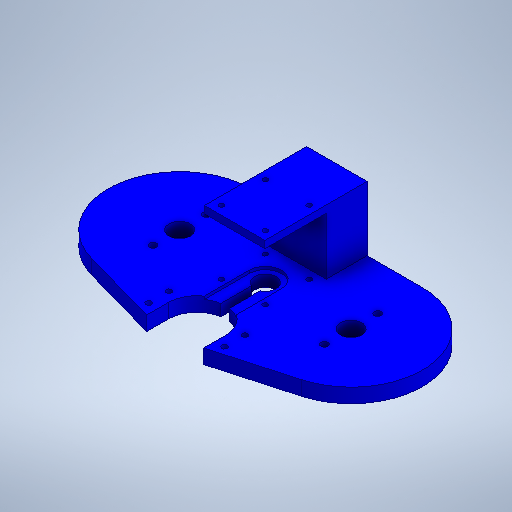
# Autodesk Inventor part: ExtruderFrame
Saved by Autodesk Inventor 2025.2 (Build 292293000, 293)
## iProperties
Created: 2025-05-30
Part Number: ExtruderFrame
Material: Generic
Document SubType Name: Modeling
Designer: Simon
Density: 1 g/cm^3
Appearance: Default(2)
Author: Simon
Autodesk Inventor part; units mm, degrees
ref_plane "YZ Plane" through (0, 0, 0) normal (1, 0, 0) x (0, 1, 0)
ref_plane "XZ Plane" through (0, 0, 0) normal (0, 1, 0) x (-1, 0, 0)
ref_plane "XY Plane" through (0, 0, 0) normal (0, 0, 1) x (1, 0, 0)
sketch "Sketch6" plane through (0, 0, 0) normal (0, 1, 0) x (-1, 0, 0)
  line L0 (60, 0) -> (-60, 0)
  circle A0 centre (0, 0) radius 30
  circle A1 centre (-60, 0) radius 50
  circle A2 centre (60, 0) radius 50
  circle A3 centre (60, 0) radius 7.5
  circle A4 centre (0, 0) radius 7.5
  circle A5 centre (-60, 0) radius 7.5
  line L1 (60, -50) -> (-60, -50)
  line L2 (-60, 18.65) -> (-60, -18.65)
  line L3 (60, 18.65) -> (60, -18.65)
  line L4 (0, -15.3795) -> (0, 15.3795)
  line L5 (15.3795, 15.3795) -> (-15.3795, 15.3795)
  line L6 (15.3795, -15.3795) -> (-15.3795, -15.3795)
  line L7 (21.15, 21.5) -> (-21.15, 21.5)
  line L8 (-21.15, 21.5) -> (-21.15, -21.5)
  line L9 (-21.15, -21.5) -> (21.15, -21.5)
  line L10 (21.15, -21.5) -> (21.15, 21.5)
  line L11 (21.15, 21.5) -> (-21.15, -21.5) construction
  line L12 (-21.15, 21.5) -> (21.15, -21.5) construction
  line L13 (21.15, -21.5) -> (-21.15, -21.5)
  line L14 (-21.15, -21.5) -> (-21.15, -50)
  line L15 (-21.15, -50) -> (21.15, -50)
  line L16 (21.15, -50) -> (21.15, -21.5)
  line L17 (7.5, 0) -> (-7.7, 0)
  line L18 (-7.7, 0) -> (-7.7, 50)
  line L19 (-7.7, 50) -> (7.5, 50)
  line L20 (7.5, 50) -> (7.5, 0)
  line L21 (3, -100) -> (-3, -100)
  line L22 (-3, -100) -> (-3, 100)
  line L23 (-3, 100) -> (3, 100)
  line L24 (3, 100) -> (3, -100)
  line L25 (3, -100) -> (-3, 100) construction
  line L26 (-3, -100) -> (3, 100) construction
  line L27 (11.25, 100) -> (-11.25, 100)
  line L28 (-11.25, 100) -> (-11.25, -100)
  line L29 (-11.25, -100) -> (11.25, -100)
  line L30 (11.25, -100) -> (11.25, 100)
  line L31 (11.25, 100) -> (-11.25, -100) construction
  line L32 (-11.25, 100) -> (11.25, -100) construction
  circle A6 centre (0, 0) radius 11.25
  line L33 (0, 0) -> (0, 48)
  circle A7 centre (0, 48) radius 20
  line L34 (73.5118, 48.1397) -> (5.4047, 67.2559)
  line L35 (-73.5118, 48.1397) -> (-5.4047, 67.2559)
  line L36 (-20, 48) -> (20, 48)
  line L37 (20, 48) -> (20, 63.1593)
  line L38 (-20, 48) -> (-20, 63.1593)
  circle A8 centre (0, 48) radius 27.5
  line L39 (0, 48) -> (-26.563, 40.8825)
  line L40 (0, 48) -> (27.5, 48) construction
  line L41 (0, 48) -> (-26.563, 55.1175)
  line L42 (0, 48) -> (26.563, 40.8825)
  line L43 (0, 48) -> (26.563, 55.1175)
  point P0 (16.6667, 24.9444)
  point P1 (-16.6667, 24.9444)
  point P2 (-7.5, 0)
  point P3 (-3, 0)
  point P4 (3, 0)
  point P5 (-21.15, -21.5)
  point P6 (21.15, -50)
  point P7 (11.25, 0)
  point P8 (3, 100)
  point P9 (-11.25, 0)
  point P10 (-11.25, 65.6152)
  point P11 (-7.7, 28.995)
  point P12 (-7.7, 29.5417)
  point P13 (-11.25, 64.5359)
  point P14 (11.25, 65.6152)
  point P15 (11.25, 64.5359)
  point P16 (7.5, 29.4595)
  point P17 (7.5, 29.0474)
  point P18 (-6.8464, 29.2083)
  point P19 (6.8464, 29.2083)
  dimension "d42" = 15
  dimension "d37" = 120
  dimension "d38" = 60
  dimension "d39" = 100
  dimension "d40" = 100
  dimension "d41" = 15
  dimension "d43" = 15
  dimension "d46" = 37.3
  dimension "d47" = 37.3
  dimension "d48" = 30.759
  dimension "d49" = 30.759
  dimension "d50" = 30.759
  dimension "d65" = 42.3
  dimension "d66" = 43
  dimension "d67" = 50
  dimension "d70" = 6
  dimension "d71" = 200
  dimension "d76" = 22.5
  dimension "d77" = 200
  dimension "d93" = 48
  dimension "d94" = 40
  dimension "d97" = 55
  dimension "d98" = 165
  constraints: 88 end point, 14 midpoint, 13 parallel, 11 point on circle, 8 centre point, 8 coincident, 7 perpendicular, 6 horizontal, 6 tangent, 5 point on line, 4 vertical, 1 equal length, 3 other
  measures "d37" distance of L0.start L0.end
  measures "d38" diameter of A0
  measures "d39" diameter of A1
  measures "d40" diameter of A2
  measures "d41" diameter of A3
  measures "d43" diameter of A5
  measures "d46" distance of L2.start L2.end
  measures "d47" distance of L3.start L3.end
  measures "d48" distance of L4.start L4.end
  measures "d49" distance of L5.start L5.end
  measures "d50" distance of L6.start L6.end
  measures "d65" distance of L9.end L8.end
  measures "d66" distance of L8.end L7.end
  measures "d67" distance of L17.end L18.end
  measures "d70" distance of L21.start L21.end
  measures "d71" distance of L21.end L22.end
  measures "d76" distance of L27.start L27.end
  measures "d77" distance of L28.end L27.end
  measures "d93" distance of L33.start L33.end
  measures "d94" diameter of A7
  measures "d97" diameter of A8
  measures "d98" angle of L39 L40
extrude "Extrusion8" add sketch "Sketch6" against normal blind 10 contours L0 A4 L22 A6 A1 | L18 A6 L22 A4 L0 | L0 A1 A6 L18 | A1 A6 L0 | L0 A6 A1 | A6 A1 L28 L5 L18 | L18 L5 L22 A6 | L28 A1 L9 A0 L8 L0 | L0 L8 A0 L7 A1 L28 | A6 A1 L28 | L28 A1 A6 | A6 L22 L6 L28 A1 | L22 A6 L4 A4 | A4 L4 A6 L22 | L18 L7 A8 L22 L5 | L5 L28 L7 L18 | L22 L5 L4 A6 | L8 A0 L0 | L0 A0 L8 | A1 L5 L28 | L28 L6 A1 | A6 L4 L6 L22 | L4 A6 L24 A4 | A4 L24 A6 L4 | L22 A8 L33 L5 | L5 A1 L7 L28 | L18 A8 L7 | L7 L28 A8 L18 | L4 L5 L24 A6 | A0 L8 L14 A1 A8 L7 | L8 L7 A0 | A0 L9 L8 | L6 L28 L9 A1 | L6 L22 L9 L28 | L6 L24 L9 L22 | A6 L24 L6 L4 | L24 A6 L20 A4 | A4 L0 A2 A6 L24 | L33 A8 L24 L5 | A8 L7 L22 | L22 L7 L33 A8 | L7 A1 A0 A8 L28 | A8 L18 A0 A7 L22 L7 | A8 L28 A0 L18 | L24 L5 L20 A6 | A0 A1 L7 | L9 A1 A0 | A0 A1 L14 L9 | L9 L28 A0 A1 | L9 L22 A0 L28 | L9 L24 A0 L22 | A6 A2 L30 L6 L24 | L20 A6 A2 L0 | L24 A8 L7 L20 L5 | L33 L7 L24 A8 | L22 A7 L33 L7 | A8 A0 L28 | L18 A7 A0 | A0 L28 A7 L18 | L20 L5 L30 A2 A6 | A1 A8 A0 | A0 L28 L1 L14 A1 | L14 L1 A1 | A0 L22 L1 L28 | L6 L30 L9 L24 | L9 L30 A0 L24 | A0 L24 L1 L22 | A6 L30 A2 | A2 L0 A6 | A2 A6 L0 | L20 L7 L30 L5 | L24 L7 A8 | L33 A7 L24 L7 | A7 A0 L22 | L22 A0 L33 A7 | A0 A8 A1 L39 A7 L28 | A2 L30 A6 | A8 A1 | L30 A2 L6 | L6 A2 L9 L30 | L9 A2 A0 L30 | A0 L30 L1 L24 | L30 L0 L10 A0 L9 A2 | L30 A2 L7 A0 L10 L0 | L30 L7 A2 L5 | L5 A2 L30 | L20 A8 L30 L7 | L7 A8 L20 | L24 A7 A0 L20 A8 L7 | L33 A0 L24 A7 | A1 L35 A8 | L9 A0 A2 | A0 A2 L16 L1 L30 | L10 A0 L0 | L0 A0 L10 | L30 A8 A0 A2 L7 | L20 A0 L30 A8 | L24 A0 A7 | L39 A8 L41 L38 A7 | L35 L38 L41 A8 | A0 L9 L16 A2 | A0 L10 L9 | A0 L10 L7 A2 A8 L16 | A0 L7 L10 | A2 A0 L7 | L30 A0 A8 | L20 A7 L30 A0 | A0 A7 L20 | L38 L41 A7 | L35 L28 A7 L41 L38 | A2 L1 L16 | A0 A8 A2 | L30 A7 L42 A8 A2 A0 | A2 A8 | A8 L34 A2 | A7 L37 L43 A8 L42 | A7 L43 L37 | L30 L34 L37 L43 A7 | A8 L43 L37 L34
hole "Hole1" at (-15.3795, 0, -15.3795) at (15.3795, 0, -15.3795) at (-15.3795, 0, 15.3795) at (15.3795, 0, 15.3795) direction (0, -1, 0) diameter 3.5 end through all
hole "Hole2" at (-60, 0, -18.65) at (-60, 0, 18.65) at (60, 0, 18.65) at (60, 0, -18.65) direction (0, -1, 0) diameter 5 end through all
extrude "Extrusion10" cut sketch "Sketch6" against normal blind 15 contours L22 A4 L4 L0 | L22 A6 L4 A4 | L22 L5 L4 A6 | L4 A4 L24 L0 | L4 A6 L24 A4 | L22 A8 L33 L5 | L4 L5 L24 A6 | L33 A8 L24 L5 | L22 L7 L33 A8 | L33 L7 L24 A8 | L22 A7 L33 L7 | L33 A7 L24 L7 | L22 A0 L33 A7 | L33 A0 L24 A7 | L22 L39 L33 A0 | L33 L42 L24 A0 | L22 L36 L39 | L43 L24 L36 | L36 L22 L41 | L36 L24 L42 | L41 L22 L19 L24 L43 | A8 L24 A7 L22 | L22 L23 L24 A8 | L22 A7 L24 L19 picked at (-2, 2.2913) picked at (-0.6788, 8.7113) picked at (2, 2.2913) picked at (0.6788, 8.7113)
extrude "Extrusion11" add sketch "Sketch6" along normal blind 45 contours L9 A1 A0 | A0 A1 L14 L9 | L9 L28 A0 A1 | L9 L22 A0 L28 | L9 L24 A0 L22 | A0 L28 L1 L14 A1 | A0 L22 L1 L28 | L9 L30 A0 L24 | A0 L24 L1 L22 | L9 A2 A0 L30 | A0 L30 L1 L24 | L9 A0 A2 | A0 A2 L16 L1 L30 | A0 L9 L16 A2
extrude "Extrusion12" cut sketch "Sketch6" against normal blind 2 contours L0 A4 L22 A6 A1 | L18 A6 L22 A4 L0 | L0 A1 A6 L18 | A1 A6 L0 | L0 A6 A1 | A4 L22 L0 | L0 L22 A4 | A6 A1 L28 L5 L18 | L18 L5 L22 A6 | L28 A1 A6 | L22 A4 L4 L0 | L0 L4 A4 L22 | L22 A6 L4 A4 | A4 L4 A6 L22 | L18 L7 A8 L22 L5 | L5 L28 L7 L18 | L22 L5 L4 A6 | L4 A4 L24 L0 | L0 L24 A4 L4 | L4 A6 L24 A4 | A4 L24 A6 L4 | L22 A8 L33 L5 | L18 A8 L7 | L7 L28 A8 L18 | L4 L5 L24 A6 | L24 A4 L0 | L0 A4 L24 | L24 A6 L20 A4 | A4 L0 A2 A6 L24 | L33 A8 L24 L5 | A8 L7 L22 | L22 L7 L33 A8 | A8 L18 A0 A7 L22 L7 | A8 L28 A0 L18 | L24 L5 L20 A6 | L20 A6 A2 L0 | L24 A8 L7 L20 L5 | L33 L7 L24 A8 | L22 A7 L33 L7 | L18 A7 A0 | A0 L28 A7 L18 | L20 L5 L30 A2 A6 | A2 L0 A6 | A2 A6 L0 | L20 L7 L30 L5 | L24 L7 A8 | L33 A7 L24 L7 | A7 A0 L22 | L22 A0 L33 A7 | A7 L18 L39 L22 A0 | A7 L28 L39 L18 | A2 L30 A6 | L20 A8 L30 L7 | L7 A8 L20 | L24 A7 A0 L20 A8 L7 | L33 A0 L24 A7 | L22 L39 L33 A0 | L39 L28 L36 L18 | L18 L36 L22 L39 | L20 A0 L30 A8 | L24 A0 A7 | L33 L42 L24 A0 | L22 L36 L39 | L36 L28 L41 L19 L18 | L18 L19 L41 L22 L36 | L20 A7 L30 A0 | A0 A7 L20 | L24 L42 L20 A7 A0 | L43 L24 L36 | L36 L22 L41 | L36 L24 L42 | L41 L22 L19 L24 L43 | A8 L22 A7 L35 L28 | L28 L27 L22 A8 | L20 L42 L30 A7 | L24 L36 L20 L42 | L24 L43 L19 L20 L36 | L41 L19 L22 | L24 L19 L43 | L28 A7 L22 L19 L41 | L35 A7 L28 | A8 L24 A7 L22 | L22 L23 L24 A8 | L20 L36 L30 L42 | L20 L19 L43 L30 L36 | L22 A7 L24 L19 | L24 A7 L30 L43 L19 | A8 L30 L34 A7 L24 | L24 L27 L30 A8 | L34 L30 A7 picked at (-11.0577, 5.3029) picked at (11.0577, 5.3029)
sketch "Sketch7" plane through (-21.15, 0, -21.5) normal (0, 0, 1) x (1, 0, 0)
  line L0 (0, 0) -> (0, 45) projected
  line L1 (42.3, 0) -> (42.3, 45) projected
  line L2 (0, 45) -> (42.3, 45)
  line L3 (42.3, 45) -> (42.3, 40)
  line L4 (42.3, 40) -> (0, 40)
  line L5 (0, 40) -> (0, 45)
  point P0 (21.15, 0)
  point P1 (0, 40)
  dimension "d80" = 5
  constraints: 8 end point, 2 parallel, 1 horizontal, 1 perpendicular, 1 point on line
  measures "d80" distance of L2.end L3.end
extrude "Extrusion13" add sketch "Sketch7" along normal blind 43
sketch "Sketch8" plane through (0, 45, 0) normal (0, 1, 0) x (1, 0, 0)
  line L0 (-15.3795, -15.3795) -> (15.3795, -15.3795)
  line L1 (15.3795, -15.3795) -> (15.3795, 15.3795)
  line L2 (15.3795, 15.3795) -> (-15.3795, 15.3795)
  line L3 (-15.3795, 15.3795) -> (-15.3795, -15.3795)
  arc A0 (3, -6.8739) -> (-3, -6.8739) centre (0, 0) ccw projected
  line L4 (-15.3795, -15.3795) -> (15.3795, 15.3795) construction
  line L5 (15.3795, -15.3795) -> (-15.3795, 15.3795) construction
  dimension "d83" = 30.759
  dimension "d84" = 30.759
  constraints: 12 end point, 2 midpoint, 2 parallel, 1 horizontal, 1 perpendicular
  measures "d83" distance of L2.end L1.end
  measures "d84" distance of L1.end L0.end
hole "Hole3" at (-15.3795, 45, -15.3795) at (15.3795, 45, -15.3795) at (15.3795, 45, 15.3795) at (-15.3795, 45, 15.3795) direction (0, -1, 0) diameter 3.5 end through all
extrude "Extrusion14" cut sketch "Sketch6" against normal through all contours A7 A0 L22 | L22 A0 L33 A7 | L33 A0 L24 A7 | L24 A0 A7 | L38 L41 A7 | L35 L28 A7 L41 L38 | A7 L43 L37 | L30 L34 L37 L43 A7
hole "Hole4" at (26.563, 0, 40.8825) at (26.563, 0, 55.1175) at (-26.563, 0, 40.8825) at (-26.563, 0, 55.1175) direction (0, -1, 0) diameter 4 end through all
body "Solid2"
